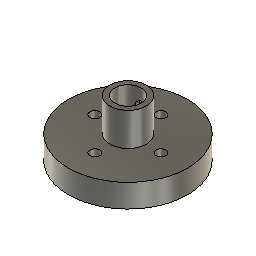
coupling (Autodesk Fusion 360 design; units mm, degrees)
part number: 2025-04-08-18-30-47-218
Autodesk Fusion 360 part; units mm, degrees
sketch "Sketch1" plane through (0, 0, 0) normal (0, 0, 1) x (1, 0, 0)
  circle A0 centre (0, 0) radius 18
  dimension "d1" = 36
  constraint coincident A0.centre origin
  measures "d1" diameter of A0
extrude "Extrude1" add sketch "Sketch1" along normal blind 7
sketch "Sketch2" plane through (0, 0, 7) normal (0, 0, 1) x (-1, 0, 0)
  circle A0 centre (0, 0) radius 18
  circle A1 centre (0, -10) radius 1.5
  circle A2 centre (10, 0) radius 1.5
  circle A3 centre (0, 10) radius 1.5
  circle A4 centre (-10, 0) radius 1.5
  dimension "d4" = 3
  dimension "d5" = 10
  dimension "d7" = 360
  constraint vertical A0.centre A1.centre
  measures "d4" diameter of A1
  measures "d5" vertical distance of A0.centre A1.centre
hole "Hole1" at (-10, 0, 7) at (0, -10, 7) at (0, 10, 7) at (10, 0, 7) direction (0, 0, -1) diameter 3 depth 300 tip angle 118
sketch "Sketch3" plane through (0, 0, 7) normal (0, 0, 1) x (-1, 0, 0)
  circle A0 centre (0, -10) radius 1.5
  circle A1 centre (10, 0) radius 1.5
  circle A2 centre (0, 10) radius 1.5
  circle A3 centre (-10, 0) radius 1.5
  circle A4 centre (0, 0) radius 18
  circle A5 centre (0, 0) radius 4
  circle A6 centre (0, 0) radius 5.5
  dimension "d11" = 8
  dimension "d12" = 1.5
  constraint concentric A4 A5
  constraint concentric A4 A6
  measures "d11" diameter of A5
  measures "d12" distance of A5 A6
extrude "Extrude2" add sketch "Sketch3" along normal blind 10 contours A6
ref_plane "WorkPlane1" through (0, 20, 0) normal (0, 1, 0) x (0, 0, 1)
sketch "Sketch4" plane through (0, 20, 0) normal (0, 1, 0) x (1, 0, 0)
  circle A0 centre (0, -12) radius 1.5
  line L0 (-5.5, -17) -> (5.5, -17)
  dimension "d16" = 5
  dimension "d17" = 3
  measures "d16" distance of A0.centre L0
  measures "d17" diameter of A0
extrude "Extrude3" cut sketch "Sketch4" against normal blind 18
fillet "Fillet1" radius 0.3 1 edges at (-1.5, 5.2915, 12)
ref_plane "WorkPlane2" through (0, 0, 17) normal (0, 0, 1) x (1, 0, 0)
sketch "Sketch5" plane through (0, 0, 17) normal (0, 0, 1) x (1, 0, 0)
  circle A0 centre (0, 0) radius 18
  constraint coincident A0.centre origin
extrude "Extrude6" cut sketch "Sketch3" against normal blind 19 contours A5
fillet "Fillet2" radius 0.5 1 edges at (3.7293, 1.4465, 0)
